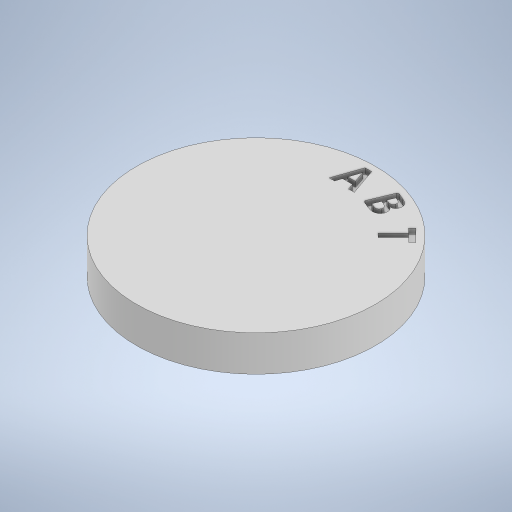
# Autodesk Inventor part: rot_th
Saved by Autodesk Inventor 2023 (Build 270158000, 158)
## iProperties
Created: 2023-05-20
Part Number: rot_th
Material: 常规
Document SubType Name: Modeling
Designer: LiuZeshu
Density: 1 g/cm^3
Appearance: 默认
Author: LiuZeshu
Autodesk Inventor part; units mm, degrees
ref_plane "YZ Plane" through (0, 0, 0) normal (1, 0, 0) x (0, 1, 0)
ref_plane "XZ Plane" through (0, 0, 0) normal (0, 1, 0) x (-1, 0, 0)
ref_plane "XY Plane" through (0, 0, 0) normal (0, 0, 1) x (1, 0, 0)
sketch "草图1" plane through (0, 0, 0) normal (0, 1, 0) x (-1, 0, 0)
  arc A0 (1.3748, -0.6) -> (-1.3748, -0.6) centre (0, 0) ccw
  line L0 (1.3748, -0.6) -> (-1.3748, -0.6)
  circle A1 centre (0, 0) radius 9
  dimension "d0" = 3
  dimension "d1" = 2.1
  dimension "d2" = 18
  constraints: 2 centre point, 2 coincident, 2 end point, 2 point on circle, 1 horizontal
  measures "d0" diameter of A0
  measures "d2" diameter of A1
extrude "拉伸1" add sketch "草图1" along normal blind 2.3
sketch "草图2" plane through (0, 2.3, 0) normal (0, 1, 0) x (1, 0, 0)
  circle A0 centre (0, 0) radius 9
  dimension "d7" = 18
  constraints: 1 centre point, 1 coincident
  measures "d7" diameter of A0
extrude "拉伸2" add sketch "草图2" along normal blind 0.4
sketch "草图3" plane through (0, 2.7, 0) normal (0, 1, 0) x (1, 0, 0)
  line L0 (0, 0) -> (0, 10.4823)
  line L1 (-0.7481, 7.9877) -> (0.7481, 7.9877) construction
  line L2 (0.7481, 7.9877) -> (0.7481, 6.5) construction
  line L3 (0.7481, 6.5) -> (-0.7481, 6.5) construction
  line L4 (-0.7481, 6.5) -> (-0.7481, 7.9877) construction
  line L5 (0, 0) -> (-4.0114, 9.6844)
  line L6 (0, 0) -> (-7.4121, 7.4121)
  line L7 (0, 0) -> (-9.6844, 4.0114)
  line L8 (0, 0) -> (-10.4823, 0)
  line L9 (0, 0) -> (-9.6844, -4.0114)
  line L10 (0, 0) -> (-7.4121, -7.4121)
  line L11 (0, 0) -> (-4.0114, -9.6844)
  line L12 (0, 0) -> (0, -10.4823)
  line L13 (0, 0) -> (4.0114, -9.6844)
  line L14 (0, 0) -> (7.4121, -7.4121)
  line L15 (0, 0) -> (9.6844, -4.0114)
  line L16 (0, 0) -> (10.4823, 0)
  line L17 (0, 0) -> (9.6844, 4.0114)
  line L18 (0, 0) -> (7.4121, 7.4121)
  line L19 (0, 0) -> (4.0114, 9.6844)
  line L20 (2.0839, 8.406) -> (4.4704, 7.4175) construction
  line L21 (4.4704, 7.4175) -> (3.6807, 5.5109) construction
  line L22 (3.6807, 5.5109) -> (1.2942, 6.4995) construction
  line L23 (1.2942, 6.4995) -> (2.0839, 8.406) construction
  line L24 (3.6829, 5.5095) -> (4.5678, 6.3944) construction
  line L25 (4.5678, 6.3944) -> (6.3944, 4.5678) construction
  line L26 (6.3944, 4.5678) -> (5.5095, 3.6829) construction
  line L27 (5.5095, 3.6829) -> (3.6829, 5.5095) construction
  line L28 (0.9024, 6.5013) -> (0.4624, 6.5013)
  line L29 (0.4624, 6.5013) -> (0.3119, 6.9554)
  line L30 (0.3119, 6.9554) -> (-0.4394, 6.9554)
  line L31 (-0.4394, 6.9554) -> (-0.5848, 6.5013)
  line L32 (-0.5848, 6.5013) -> (-0.9917, 6.5013)
  line L33 (-0.9917, 6.5013) -> (-0.2953, 8.5089)
  line L34 (-0.2953, 8.5089) -> (0.2034, 8.5089)
  line L35 (0.2034, 8.5089) -> (0.9024, 6.5013)
  line L36 (-0.0657, 8.1173) -> (-0.067, 8.1173)
  line L37 (-0.067, 8.1173) -> (-0.3501, 7.2679)
  line L38 (-0.3501, 7.2679) -> (0.2175, 7.2679)
  line L39 (0.2175, 7.2679) -> (-0.0657, 8.1173)
  spline S0 degree 2 poles (3.3789, 6.2876) (3.3379, 6.1886) (3.2173, 6.0508) (3.0711, 5.9678) (2.9015, 5.9317) (2.7179, 5.9415) (2.5252, 5.9896) (2.4144, 6.0355) knots 0 0 0 1 2 3 4 5 6 6 6
  line L40 (2.4144, 6.0355) -> (1.923, 6.239)
  spline S1 degree 2 poles (1.923, 6.239) (1.8758, 6.2585) (1.8352, 6.3403) (1.8615, 6.4039) knots 0 0 0 1 2 2 2
  line L41 (1.8615, 6.4039) -> (2.5317, 8.0219)
  spline S2 degree 2 poles (2.5317, 8.0219) (2.5576, 8.0844) (2.6441, 8.1134) (2.6913, 8.0939) knots 0 0 0 1 2 2 2
  line L42 (2.6913, 8.0939) -> (3.1556, 7.9015)
  spline S3 degree 2 poles (3.1556, 7.9015) (3.3253, 7.8312) (3.5375, 7.6771) (3.6502, 7.4923) (3.6618, 7.2804) (3.6115, 7.1591) knots 0 0 0 1 2 3 4 4 4
  spline S4 degree 2 poles (3.6115, 7.1591) (3.5837, 7.0919) (3.5007, 6.9882) (3.3947, 6.9189) (3.2675, 6.8819) (3.1969, 6.8848) knots 0 0 0 1 2 3 4 4 4
  spline S5 degree 2 poles (3.1969, 6.8848) (3.27, 6.838) (3.3723, 6.7114) (3.4249, 6.5585) (3.418, 6.3819) (3.3789, 6.2876) knots 0 0 0 1 2 3 4 4 4
  spline S6 degree 2 poles (2.9847, 6.4357) (3.0115, 6.5005) (3.0099, 6.6199) (2.9562, 6.7236) (2.8434, 6.8145) (2.7409, 6.857) knots 0 0 0 1 2 3 4 4 4
  line L43 (2.7409, 6.857) -> (2.5181, 6.9493)
  line L44 (2.5181, 6.9493) -> (2.2995, 6.4213)
  line L45 (2.2995, 6.4213) -> (2.5705, 6.3091)
  spline S7 degree 2 poles (2.5705, 6.3091) (2.6495, 6.2764) (2.7699, 6.2638) (2.8745, 6.2964) (2.9593, 6.3744) (2.9847, 6.4357) knots 0 0 0 1 2 3 4 4 4
  spline S8 degree 2 poles (3.2182, 7.2695) (3.2416, 7.3261) (3.2441, 7.4286) (3.199, 7.5163) (3.108, 7.5899) (3.0207, 7.626) knots 0 0 0 1 2 3 4 4 4
  line L46 (3.0207, 7.626) -> (2.831, 7.7046)
  line L47 (2.831, 7.7046) -> (2.6319, 7.2238)
  line L48 (2.6319, 7.2238) -> (2.8416, 7.1369)
  spline S9 degree 2 poles (2.8416, 7.1369) (2.9229, 7.1033) (3.0369, 7.1016) (3.1283, 7.1425) (3.1972, 7.2188) (3.2182, 7.2695) knots 0 0 0 1 2 3 4 4 4
  line L49 (6.2151, 5.2862) -> (5.8923, 5.6091)
  line L50 (5.8923, 5.6091) -> (4.7387, 4.4555)
  line L51 (4.7387, 4.4555) -> (4.4501, 4.7423)
  line L52 (4.4501, 4.7423) -> (5.6027, 5.895)
  line L53 (5.6027, 5.895) -> (5.2817, 6.216)
  line L54 (5.2817, 6.216) -> (5.5522, 6.4866)
  line L55 (5.5522, 6.4866) -> (6.4839, 5.5549)
  line L56 (6.4839, 5.5549) -> (6.2151, 5.2862)
  point P0 (0, 7.9877)
  point P1 (0, 7.9877)
  point P2 (-3.0568, 7.3797)
  point P3 (-3.0568, 7.3797)
  point P4 (-5.6481, 5.6481)
  point P5 (-5.6481, 5.6481)
  point P6 (-7.3797, 3.0568)
  point P7 (-7.3797, 3.0568)
  point P8 (-7.9877, 0)
  point P9 (-7.9877, 0)
  point P10 (-7.3797, -3.0568)
  point P11 (-7.3797, -3.0568)
  point P12 (-5.6481, -5.6481)
  point P13 (-5.6481, -5.6481)
  point P14 (-3.0568, -7.3797)
  point P15 (-3.0568, -7.3797)
  point P16 (0, -7.9877)
  point P17 (0, -7.9877)
  point P18 (3.0568, -7.3797)
  point P19 (3.0568, -7.3797)
  point P20 (5.6481, -5.6481)
  point P21 (5.6481, -5.6481)
  point P22 (7.3797, -3.0568)
  point P23 (7.3797, -3.0568)
  point P24 (7.9877, 0)
  point P25 (7.9877, 0)
  point P26 (7.3797, 3.0568)
  point P27 (7.3797, 3.0568)
  point P28 (5.6481, 5.6481)
  point P29 (5.6481, 5.6481)
  point P30 (3.0568, 7.3797)
  point P31 (3.0568, 7.3797)
  point P32 (1.625, 8.5961)
  point P33 (3.2772, 7.9117)
  point P34 (2.6779, 8.2844)
  point P35 (5.4811, 5.4811)
  dimension "d17" = 360
  dimension "d19" = 6.5
  dimension "d20" = 6.5
  dimension "d21" = 6.5
  constraints: 32 end point, 21 point on line, 4 midpoint, 3 coincident, 3 perpendicular, 1 vertical, 85 other
  measures "d19" distance from line of L0.start L3
  measures "d20" distance from line of L0.start L22
  measures "d21" distance from line of L0.start L27
extrude "拉伸3" cut sketch "草图3" against normal blind 0.4 contours L30 L31 L32 L33 L34 L0 L39 L37 L38 | L0 L38 L39 L34 L35 L28 L29 L30 | L51 L52 L53 L54 L55 L18 | L18 L55 L56 L49 L50 L51 | S0 L40 S1 L41 S2 L42 S3 L19 S8 L46 L47 L48 S9 S6 L43 L44 L45 S7 | L19 S7 S6 S9 S8 S3 S4 S5 S0
